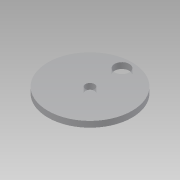
# Autodesk Inventor part: Gland Disk3
Saved by Autodesk Inventor 2015 (Build 190159000, 159)
## iProperties
Created: 2011-09-29
Part Number: Gland Disk3
Document SubType Name: Modeling
Designer: user
Density: 1 g/cm^3
Material: Generic
Appearance: Polycarbonate - Clear
Author: user
Autodesk Inventor part; units mm, degrees
ref_plane "YZ Plane" through (0, 0, 0) normal (1, 0, 0) x (0, 1, 0)
ref_plane "XZ Plane" through (0, 0, 0) normal (0, 1, 0) x (-1, 0, 0)
ref_plane "XY Plane" through (0, 0, 0) normal (0, 0, 1) x (1, 0, 0)
sketch "Sketch1" plane through (0, 0, 0) normal (0, 0, 1) x (1, 0, 0)
  circle A0 centre (0, 0) radius 42.75
  circle A1 centre (0, 0) radius 4.59
  circle A2 centre (0, 32.5) radius 7.5
  dimension "d0" = 85.5
  dimension "d1" = 9.18
  dimension "d4" = 15
  dimension "d6" = 32.5
  constraints: 3 centre point, 2 coincident, 1 vertical alignment
  measures "d0" diameter of A0
  measures "d1" diameter of A1
  measures "d4" diameter of A2
  measures "d6" distance of A1.centre A2.centre
extrude "Extrusion2" add sketch "Sketch1" along normal blind 6
body "Solid2"
